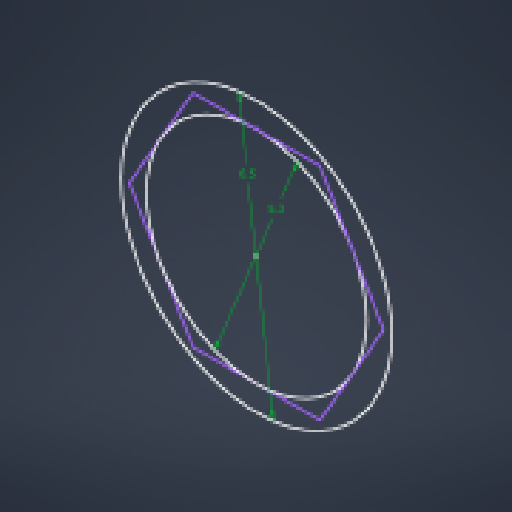
# Autodesk Inventor part: 12.55mm Slim Spacer
Saved by Autodesk Inventor 2023 (Build 270158000, 158)
## iProperties
Created: 2022-11-13
Part Number: 12.55mm Slim Spacer
Material: Generic
Document SubType Name: Modeling
Designer: izack
Density: 1 g/cm^3
Appearance: Default
Author: izack
Autodesk Inventor part; units mm, degrees
ref_plane "YZ Plane" through (0, 0, 0) normal (1, 0, 0) x (0, 1, 0)
ref_plane "XZ Plane" through (0, 0, 0) normal (0, 1, 0) x (-1, 0, 0)
ref_plane "XY Plane" through (0, 0, 0) normal (0, 0, 1) x (1, 0, 0)
sketch "Sketch1" plane through (0, 0, 0) normal (0, 0, 1) x (1, 0, 0)
  circle A0 centre (0, 0) radius 2.65
  line L0 (1.53, 2.65) -> (3.06, 0)
  line L1 (3.06, 0) -> (1.53, -2.65)
  line L2 (1.53, -2.65) -> (-1.53, -2.65)
  line L3 (-1.53, -2.65) -> (-3.06, 0)
  line L4 (-3.06, 0) -> (-1.53, 2.65)
  line L5 (-1.53, 2.65) -> (1.53, 2.65)
  circle A1 centre (0, 0) radius 3.25
  point P0 (0, 2.65)
  dimension "d0" = 5.3
  dimension "d1" = 6.5
  constraints: 12 end point, 3 coincident, 1 centre point, 1 midpoint, 1 vertical alignment, 15 other
  measures "d1" diameter of A1
ref_plane "Work Plane1" through (-4.5387, -4.5387, 12.5) normal (0, 0, -1) x (0.2174352, 0.9760748, 0)
extrude "Extrusion1" add sketch "Sketch1" along normal up to surface (12.5 mm away)
body "Solid1"
